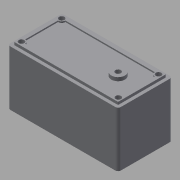
# Autodesk Inventor part: housing
Saved by Autodesk Inventor 2016 (Build 200138000, 138)
## iProperties
Created: 2013-07-12
Part Number: housing
Material: PET Plastic
Document SubType Name: Modeling
Designer: Maurice
Density: 1.541 g/cm^3
Appearance: Polycarbonate - Clear
Mass: 8.58132 g
Surface Area: 67.7931 cm^2
Volume: 5.56867 cm^3
Author: Maurice
Autodesk Inventor part; units mm, degrees
ref_plane "YZ Plane" through (0, 0, 0) normal (1, 0, 0) x (0, 1, 0)
ref_plane "XZ Plane" through (0, 0, 0) normal (0, 1, 0) x (-1, 0, 0)
ref_plane "XY Plane" through (0, 0, 0) normal (0, 0, 1) x (1, 0, 0)
sketch "Sketch1" plane through (0, 0, 0) normal (0, 1, 0) x (-1, 0, 0)
  line L0 (20.38, 10.015) -> (-20.38, 10.015)
  line L1 (-20.38, 10.015) -> (-20.38, -10.015)
  line L2 (-20.38, -10.015) -> (20.38, -10.015)
  line L3 (20.38, -10.015) -> (20.38, 10.015)
  line L4 (20.38, 10.015) -> (-20.38, -10.015) construction
  line L5 (-20.38, 10.015) -> (20.38, -10.015) construction
  point P0 (0, 0)
  dimension "d0" = 40.76
  dimension "d1" = 20.03
  constraints: 12 end point, 2 midpoint, 2 parallel, 1 horizontal, 1 perpendicular
  measures "d0" distance of L2.end L1.end
  measures "d1" distance of L1.end L0.end
extrude "Extrusion1" add sketch "Sketch1" along normal blind 21.3
sketch "Sketch2" plane through (0, 21.3, 0) normal (0, 1, 0) x (1, 0, 0)
  line L0 (-20.38, -10.015) -> (20.38, -10.015) projected
  line L1 (20.38, -10.015) -> (20.38, 10.015) projected
  line L2 (20.38, 10.015) -> (-20.38, 10.015) projected
  line L3 (-20.38, 10.015) -> (-20.38, -10.015) projected
  line L4 (-19.23, 8.865) -> (19.23, 8.865)
  line L5 (19.23, 8.865) -> (19.23, -8.865)
  line L6 (19.23, -8.865) -> (-19.23, -8.865)
  line L7 (-19.23, -8.865) -> (-19.23, 8.865)
  point P0 (0, 0)
  dimension "d4" = 1.15
  constraints: 8 end point, 3 other
  measures "d4" distance between parallel lines of L2 L4
extrude "Extrusion2" cut sketch "Sketch2" against normal blind 1
sketch "Sketch3" plane through (0, 21.3, 0) normal (0, 1, 0) x (1, 0, 0)
  line L0 (-19.23, 8.865) -> (-19.23, -8.865) projected
  line L1 (19.23, 8.865) -> (-19.23, 8.865) projected
  point P0 (0, 0)
  point P1 (-17.875, 7.42)
  point P2 (17.875, 7.42)
  point P3 (-17.875, -7.42)
  point P4 (17.875, -7.42)
  dimension "d7" = 17.875
  dimension "d8" = 7.42
  dimension "d11" = 35.75
  dimension "d14" = 14.84
  constraints: 1 horizontal, 1 vertical, 3 other
  measures "d7" horizontal distance of point (0, 0) point (-17.875, 7.42)
  measures "d8" vertical distance of point (0, 0) point (-17.875, 7.42)
  measures "d11" distance of point (-17.875, 7.42) point (17.875, 7.42)
  measures "d14" distance of point (-17.875, 7.42) point (-17.875, -7.42)
hole "Hole1" at (-17.875, 21.3, -7.42) at (17.875, 21.3, -7.42) at (-17.875, 21.3, 7.42) at (17.875, 21.3, 7.42) direction (0, -1, 0) diameter 2 end through all
shell "Shell1" thickness 1.75 removed faces 1 at (5.6467, 0, 2.3551)
sketch "Sketch5" plane through (0, 0, 0) normal (0, -1, 0) x (1, 0, 0)
  line L0 (-18.63, -4.7757) -> (-18.63, 4.7757) projected
  arc A0 (-18.63, 4.7757) -> (-15.258, 8.265) centre (-17.875, 7.42) ccw projected
  line L1 (-15.258, 8.265) -> (15.258, 8.265) projected
  arc A1 (15.258, 8.265) -> (18.63, 4.7757) centre (17.875, 7.42) ccw projected
  line L2 (18.63, 4.7757) -> (18.63, -4.7757) projected
  arc A2 (18.63, -4.7757) -> (15.258, -8.265) centre (17.875, -7.42) ccw projected
  line L3 (15.258, -8.265) -> (-15.258, -8.265) projected
  arc A3 (-15.258, -8.265) -> (-18.63, -4.7757) centre (-17.875, -7.42) ccw projected
  circle A4 centre (-17.875, 7.42) radius 1 projected
  circle A5 centre (-17.875, -7.42) radius 1 projected
  circle A6 centre (17.875, -7.42) radius 1 projected
  circle A7 centre (17.875, 7.42) radius 1 projected
  line L4 (-20.38, 10.015) -> (20.38, 10.015) projected
  line L5 (-20.38, -10.015) -> (-20.38, 10.015) projected
  line L6 (20.38, -10.015) -> (-20.38, -10.015) projected
  line L7 (20.38, 10.015) -> (20.38, -10.015) projected
  line L8 (19.38, 9.015) -> (-19.38, 9.015)
  line L9 (-19.38, 9.015) -> (-19.38, -9.015)
  line L10 (-19.38, -9.015) -> (19.38, -9.015)
  line L11 (19.38, -9.015) -> (19.38, 9.015)
  point P0 (0, 0)
  dimension "d25" = 1
  constraints: 8 end point, 3 other
  measures "d25" distance between parallel lines of L4 L8
extrude "Extrusion3" cut sketch "Sketch5" against normal blind 0.53 contours L11 L10 L9 L8
fillet "Fillet1" radius 1 4 edges at (-20.38, 10.15, 10.015) (20.38, 10.15, 10.015) (20.38, 10.15, -10.015) (-20.38, 10.15, -10.015)
sketch "Sketch6" plane through (0, 21.3, 0) normal (0, 1, 0) x (1, 0, 0)
  circle A0 centre (-17.875, -7.42) radius 1 projected
  circle A1 centre (-17.875, 7.42) radius 1 projected
  circle A2 centre (17.875, 7.42) radius 1 projected
  circle A3 centre (17.875, -7.42) radius 1 projected
  line L0 (19.23, 8.865) -> (-19.23, 8.865) projected
  line L1 (-17.875, 6.065) -> (-17.875, -6.065)
  line L2 (-16.52, -7.42) -> (16.52, -7.42)
  line L3 (17.875, -6.065) -> (17.875, 6.065)
  line L4 (16.52, 7.42) -> (-16.52, 7.42)
  arc A4 (-17.875, 6.065) -> (-16.52, 7.42) centre (-17.875, 7.42) ccw
  arc A5 (-16.52, -7.42) -> (-17.875, -6.065) centre (-17.875, -7.42) ccw
  arc A6 (17.875, -6.065) -> (16.52, -7.42) centre (17.875, -7.42) ccw
  arc A7 (16.52, 7.42) -> (17.875, 6.065) centre (17.875, 7.42) ccw
  point P0 (0, 0)
  constraints: 8 end point, 8 point on circle, 4 centre point, 4 coincident, 4 perpendicular
extrude "Extrusion4" cut sketch "Sketch6" against normal blind 0.5 contours A4 L4 A7 L3 A6 L2 A5 L1
sketch "Sketch7" plane through (0, 20.8, 0) normal (0, 1, 0) x (1, 0, 0)
  line L0 (20.38, 9.015) -> (20.38, -9.015) construction
  circle A0 centre (10.38, 0) radius 2.5
  point P0 (0, 0)
  dimension "d31" = 5
  dimension "d32" = 10
  constraints: 1 centre point, 1 horizontal alignment
  measures "d31" diameter of A0
  measures "d32" distance from line of L0 A0.centre
extrude "Extrusion5" add sketch "Sketch7" along normal blind 1.3
hole "Hole2" at (10.38, 22.1, 0) direction (0, -1, 0) diameter 2 end through all
fillet "Fillet2" radius 0.2 4 edges at (-19.23, 20.8, 8.865) (-19.23, 20.8, -8.865) (19.23, 20.8, 8.865) (19.23, 20.8, -8.865)
equation "\"d11\" = 2 * d7"
equation "\"d14\" = 2 * d8"
body "Solid1"
